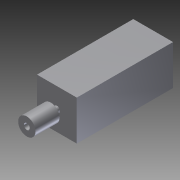
# Autodesk Inventor part: Big stepper
Saved by Autodesk Inventor 2012 (Build 160160000, 160)
## iProperties
Created: 2013-05-10
Part Number: Big stepper
Material: Default
Document SubType Name: Modeling
Designer: Fabian
Density: 1 g/cm^3
Author: Fabian
Autodesk Inventor part; units mm, degrees
ref_plane "YZ Plane" through (0, 0, 0) normal (1, 0, 0) x (0, 1, 0)
ref_plane "XZ Plane" through (0, 0, 0) normal (0, 1, 0) x (-1, 0, 0)
ref_plane "XY Plane" through (0, 0, 0) normal (0, 0, 1) x (1, 0, 0)
sketch "Sketch1" plane through (0, 0, 0) normal (0, 0, 1) x (1, 0, 0)
  line L0 (-5.8741, 27.1165) -> (36.1375, 27.1165)
  line L1 (36.1375, 27.1165) -> (36.1375, -14.8951)
  line L2 (36.1375, -14.8951) -> (-5.8741, -14.8951)
  line L3 (-5.8741, -14.8951) -> (-5.8741, 27.1165)
  point P0 (0, 0)
  dimension "d0" = 42.0116
  dimension "d1" = 42.0116
  constraints: 8 end point, 2 parallel, 1 horizontal, 1 perpendicular
  measures "d0" distance of L2.end L0.start
  measures "d1" distance of L1.end L2.end
extrude "Extrusion1" add sketch "Sketch1" along normal blind 101.6
sketch "Sketch2" plane through (0, 0, 101.6) normal (0, 0, 1) x (1, 0, 0)
  circle A0 centre (15.1317, 6.1107) radius 3.1463
  point P0 (0, 0)
  constraints: 1 centre point
extrude "Extrusion2" add sketch "Sketch2" along normal blind 6.35
sketch "Sketch3" plane through (15.1317, 6.1107, 107.95) normal (0, 0, 1) x (1, 0, 0)
  circle A0 centre (0, 0) radius 3.1463 projected
  circle A1 centre (0, 0) radius 9.1838
  point P0 (-15.1317, -6.1107)
  constraints: 1 centre point, 1 coincident
extrude "Extrusion3" add sketch "Sketch3" along normal blind 25.4
equation "\"d1\" = d0"
body "Solid1"
